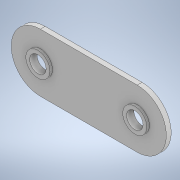
# Autodesk Inventor part: Belt Retaining Guide
Saved by Autodesk Inventor 2022 (Build 260153000, 153)
## iProperties
Created: 2021-10-06
Part Number: Belt Retaining Guide
Material: Generic
Document SubType Name: Modeling
Designer: nicol
Density: 1 g/cm^3
Appearance: Default
Author: nicol
Autodesk Inventor part; units mm, degrees
ref_plane "YZ Plane" through (0, 0, 0) normal (1, 0, 0) x (0, 1, 0)
ref_plane "XZ Plane" through (0, 0, 0) normal (0, 1, 0) x (-1, 0, 0)
ref_plane "XY Plane" through (0, 0, 0) normal (0, 0, 1) x (1, 0, 0)
sketch "Sketch1" plane through (0, 0, 0) normal (0, 0, 1) x (1, 0, 0)
  line L0 (-10, 0) -> (10, 0) construction
  line L1 (-10, -6) -> (10, -6)
  line L2 (10, 6) -> (-10, 6)
  arc A0 (-10, 6) -> (-10, -6) centre (-10, 0) ccw
  arc A1 (10, -6) -> (10, 6) centre (10, 0) ccw
  circle A2 centre (-10, 0) radius 1.7
  circle A3 centre (10, 0) radius 1.7
  point P0 (0, 0)
  point P1 (0, 0)
  dimension "d0" = 20
  dimension "d1" = 6
  dimension "d2" = 3.4
  constraints: 8 end point, 4 centre point, 4 point on circle, 4 tangent, 3 coincident, 1 equal radius, 1 horizontal, 1 midpoint, 1 parallel
  measures "d0" distance of L0.start L0.end
  measures "d1" radius of A0
  measures "d2" diameter of A2
extrude "Extrusion1" add sketch "Sketch1" along normal blind 1
sketch "Sketch2" plane through (0, 0, 1) normal (0, 0, 1) x (1, 0, 0)
  circle A0 centre (10, 0) radius 1.7 projected
  circle A1 centre (10, 0) radius 2.5
  circle A2 centre (-10, 0) radius 1.7 projected
  circle A3 centre (-10, 0) radius 2.5
  point P0 (0, 0)
  dimension "d5" = 5
  dimension "d6" = 5
  constraints: 2 centre point, 2 coincident
  measures "d5" diameter of A1
  measures "d6" diameter of A3
extrude "Extrusion2" add sketch "Sketch2" along normal blind 0.5
body "Solid1"
